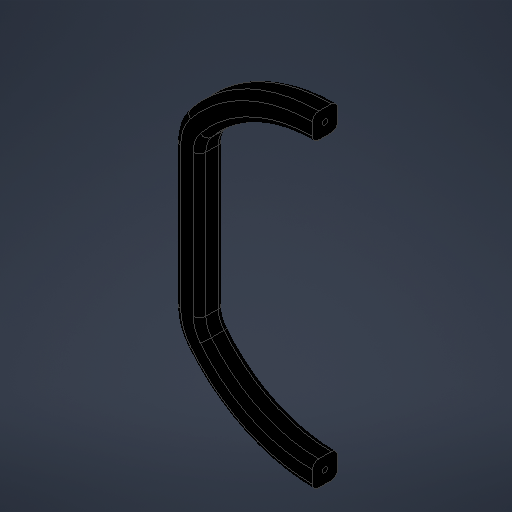
# Autodesk Inventor part: Handle
Saved by Autodesk Inventor 2026.1 (Build 301233020, 233B)
## iProperties
Created: 2025-12-04
Part Number: Handle
Material: Generic
Document SubType Name: Modeling
Designer: Bahaa
Density: 1 g/cm^3
Appearance: Default
Author: Bahaa
Autodesk Inventor part; units mm, degrees
ref_plane "YZ Plane" through (0, 0, 0) normal (1, 0, 0) x (0, 1, 0)
ref_plane "XZ Plane" through (0, 0, 0) normal (0, 1, 0) x (-1, 0, 0)
ref_plane "XY Plane" through (0, 0, 0) normal (0, 0, 1) x (1, 0, 0)
sketch "Sketch1" plane through (0, 0, 0) normal (0, 1, 0) x (-1, 0, 0)
  arc A0 (0, -120) -> (0, 120) centre (0, 0) ccw construction
  arc A1 (0, -110) -> (0, 110) centre (0, 0) ccw
  arc A2 (0, -130) -> (0, 130) centre (0, 0) ccw
  line L0 (0, 130) -> (0, 110)
  line L1 (0, -110) -> (0, -130)
  line L2 (0, 130) -> (0, -130)
  line L3 (100, 83.0662) -> (100, -83.0662)
  line L4 (90, 93.8083) -> (90, -93.8083)
  line L5 (110, 69.282) -> (110, -69.282)
  point P0 (90, 63.2456)
  point P1 (90, -63.2456)
  dimension "d16" = 120
  dimension "d17" = 10
  dimension "d18" = 10
  dimension "d19" = 20
  dimension "d20" = 20
  dimension "d21" = 0
  dimension "d25" = 10
  dimension "d26" = 10
  dimension "d27" = 110
  dimension "d28" = 110
  constraints: 12 end point, 12 point on circle, 3 centre point, 3 coincident, 3 vertical, 1 collinear, 1 parallel
  measures "d16" radius of A0
  measures "d17" radial gap between concentric circles of A1 A0
  measures "d18" radial gap between concentric circles of A0 A2
  measures "d19" distance of L1.start L1.end
  measures "d20" distance of L0.start L0.end
  measures "d21" distance from line of A0.end L0
  measures "d25" distance between parallel lines of L3 L4
  measures "d26" distance between parallel lines of L5 L3
  measures "d27" distance between parallel lines of L5 L0
  measures "d28" distance from line of A0.start L5
extrude "Extrusion1" add sketch "Sketch1" along normal blind 20 contours A1 L4 A2 L1 | L4 A1 L3 | A1 L3 A2 L4 | L0 A2 L4 A1 | L3 A1 | A1 L5 A2 L3 | L4 A2 L3 A1 | A1 L3 A2 L5
fillet "Fillet1" radius 20 2 edges at (-90, 10, -63.2456) (-90, 10, 63.2456)
fillet "Fillet2" radius 40 2 edges at (-110, 10, 69.282) (-110, 10, -69.282)
fillet "Fillet3" radius 5 20 edges at (-107.7124, 20, 69.9019) (-110, 20, 0) (-107.7124, 20, -69.9019) (-56.0254, 20, -117.308) (-56.0254, 20, 117.308) (-107.7124, 0, 69.9019) (-110, 0, 0) (-107.7124, 0, -69.9019) (-56.0254, 0, -117.308) (-56.0254, 0, 117.308) (-88.8562, 20, 63.2352) (-90, 20, 0) (-88.8562, 20, -63.2352) (-47.4061, 20, -99.2606) (-47.4061, 20, 99.2606) (-88.8562, 0, 63.2352) (-90, 0, 0) (-88.8562, 0, -63.2352) (-47.4061, 0, -99.2606) (-47.4061, 0, 99.2606)
sketch "Sketch2" plane through (0, 0, 125) normal (1, 0, 0) x (0, 0, -1)
  arc A0 (10, 0) -> (15, 5) centre (10, 5) ccw projected
  line L0 (15, 5) -> (15, 15) projected
  arc A1 (15, 15) -> (10, 20) centre (10, 15) ccw projected
  line L1 (0, 20) -> (10, 20) projected
  arc A2 (0, 20) -> (-5, 15) centre (0, 15) ccw projected
  line L2 (-5, 5) -> (-5, 15) projected
  arc A3 (-5, 5) -> (0, 0) centre (0, 5) ccw projected
  line L3 (0, 0) -> (10, 0) projected
  arc A4 (235, 5) -> (240, 0) centre (240, 5) ccw projected
  line L4 (240, 0) -> (250, 0) projected
  arc A5 (250, 0) -> (255, 5) centre (250, 5) ccw projected
  line L5 (255, 5) -> (255, 15) projected
  arc A6 (255, 15) -> (250, 20) centre (250, 15) ccw projected
  line L6 (240, 20) -> (250, 20) projected
  arc A7 (240, 20) -> (235, 15) centre (240, 15) ccw projected
  line L7 (235, 5) -> (235, 15) projected
  line L8 (245, 0) -> (245, 10) construction
  line L9 (235, 5) -> (235, 15) projected
  line L10 (235, 10) -> (245, 10) construction
  line L11 (125, 0) -> (125, 20) construction
  line L12 (181.5685, 20) -> (68.4315, 20) construction
  point P0 (5, 10)
  constraints: 6 end point, 3 midpoint, 1 coincident, 1 perpendicular, 1 symmetric about line, 1 vertical
hole "Hole1" at (0, 10, -120) at (0, 10, 120) direction (-1, 0, 0) diameter 4.2 depth 6
equation "\"d18\" = d17"
equation "\"d19\" = 2 * d17"
equation "\"d20\" = 2 * d17"
equation "\"d25\" = d17"
equation "\"d26\" = d17"
equation "\"d28\" = d27"
equation "\"d29\" = 2 * d17"
body "Solid1"
